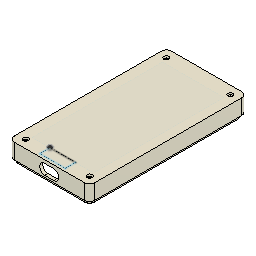
hk-case (Autodesk Fusion 360 design; units mm, degrees)
Autodesk Fusion 360 part; units mm, degrees
sketch "Base" plane through (0, 0, 0) normal (0, 1, 0) x (1, 0, 0)
  line L0 (26, -60) -> (-26, -60)
  line L1 (-30, -56) -> (-30, 56)
  line L2 (-26, 60) -> (26, 60)
  line L3 (30, 56) -> (30, -56)
  line L4 (30, -60) -> (-30, 60) construction
  line L5 (-30, -60) -> (30, 60) construction
  arc A0 (-26, 60) -> (-30, 56) centre (-26, 56) ccw
  arc A1 (30, 56) -> (26, 60) centre (26, 56) ccw
  arc A2 (-30, -56) -> (-26, -60) centre (-26, -56) ccw
  arc A3 (26, -60) -> (30, -56) centre (26, -56) ccw
  circle A4 centre (0, 0) radius 7.5
  line L6 (27.5, -61.5) -> (-27.5, -61.5)
  line L7 (-31.5, -57.5) -> (-31.5, 57.5)
  line L8 (-27.5, 61.5) -> (27.5, 61.5)
  line L9 (31.5, 57.5) -> (31.5, -57.5)
  line L10 (31.5, -61.5) -> (-31.5, 61.5) construction
  line L11 (-31.5, -61.5) -> (31.5, 61.5) construction
  arc A5 (-27.5, 61.5) -> (-31.5, 57.5) centre (-27.5, 57.5) ccw
  arc A6 (31.5, 57.5) -> (27.5, 61.5) centre (27.5, 57.5) ccw
  arc A7 (-31.5, -57.5) -> (-27.5, -61.5) centre (-27.5, -57.5) ccw
  arc A8 (27.5, -61.5) -> (31.5, -57.5) centre (27.5, -57.5) ccw
  circle A9 centre (-25, -55) radius 2.5
  circle A10 centre (25, -55) radius 2.5
  circle A11 centre (25, 55) radius 2.5
  circle A12 centre (-25, 55) radius 2.5
  circle A13 centre (-25, -55) radius 1.75
  circle A14 centre (25, -55) radius 1.75
  circle A15 centre (25, 55) radius 1.75
  circle A16 centre (-25, 55) radius 1.75
  circle A17 centre (-25, -55) radius 1
  circle A18 centre (25, -55) radius 1
  circle A19 centre (25, 55) radius 1
  circle A20 centre (-25, 55) radius 1
  circle A21 centre (-25, -55) radius 2
  circle A22 centre (25, -55) radius 2
  circle A23 centre (25, 55) radius 2
  circle A24 centre (-25, 55) radius 2
  line L12 (25, 59) -> (-25, 59)
  line L13 (-29, 55) -> (-29, -55)
  line L14 (-25, -59) -> (25, -59)
  line L15 (29, -55) -> (29, 55)
  line L16 (29, 59) -> (-29, -59) construction
  line L17 (-29, 59) -> (29, -59) construction
  arc A25 (25, -59) -> (29, -55) centre (25, -55) ccw
  arc A26 (-29, -55) -> (-25, -59) centre (-25, -55) ccw
  arc A27 (29, 55) -> (25, 59) centre (25, 55) ccw
  arc A28 (-25, 59) -> (-29, 55) centre (-25, 55) ccw
  dimension "d1" = 60
  dimension "d2" = 120
  dimension "d11" = 4
  dimension "d12" = 4
  dimension "d13" = 4
  dimension "d14" = 4
  dimension "d15" = 15
  dimension "d18" = 63
  dimension "d19" = 123
  dimension "d20" = 4
  dimension "d21" = 4
  dimension "d22" = 4
  dimension "d23" = 4
  dimension "d30" = 5
  dimension "d31" = 5
  dimension "d32" = 5
  dimension "d33" = 5
  dimension "d34" = 3.5
  dimension "d35" = 3.5
  dimension "d36" = 3.5
  dimension "d37" = 3.5
  dimension "d38" = 2
  dimension "d39" = 2
  dimension "d40" = 2
  dimension "d41" = 4
  dimension "d42" = 4
  dimension "d43" = 4
  dimension "d44" = 4
  dimension "d65" = 58
  dimension "d66" = 118
  dimension "d67" = 4
  dimension "d68" = 4
  dimension "d69" = 4
  dimension "d70" = 4
  constraint horizontal L0
  constraint perpendicular L0 L1
  constraint parallel L0 L2
  constraint parallel L1 L3
  constraint coincident L4 A4.centre
  constraint coincident L5 A4.centre
  constraint coincident A4.centre origin
  constraint coincident L4.end L2
  constraint coincident L4.end L1
  constraint tangent L2 A0
  constraint tangent L1 A0
  constraint coincident L5.end L2
  constraint coincident L5.end L3
  constraint tangent L2 A1
  constraint tangent L3 A1
  constraint coincident L5.start L1
  constraint coincident L5.start L0
  constraint tangent L1 A2
  constraint tangent L0 A2
  constraint coincident L4.start L0
  constraint coincident L4.start L3
  constraint tangent L0 A3
  constraint tangent L3 A3
  constraint horizontal L6
  constraint perpendicular L6 L7
  constraint parallel L6 L8
  constraint parallel L7 L9
  constraint coincident L10 A4.centre
  constraint coincident L11 A4.centre
  constraint coincident L10.end L8
  constraint coincident L10.end L7
  constraint tangent L8 A5
  constraint tangent L7 A5
  constraint coincident L11.end L8
  constraint coincident L11.end L9
  constraint tangent L8 A6
  constraint tangent L9 A6
  constraint coincident L11.start L7
  constraint coincident L11.start L6
  constraint tangent L7 A7
  constraint tangent L6 A7
  constraint coincident L10.start L6
  constraint coincident L10.start L9
  constraint tangent L6 A8
  constraint tangent L9 A8
  constraint concentric A9 A13
  constraint concentric A10 A14
  constraint concentric A11 A15
  constraint concentric A12 A16
  constraint concentric A9 A17
  constraint concentric A14 A18
  constraint concentric A11 A19
  constraint concentric A16 A20
  constraint concentric A13 A21
  constraint concentric A10 A22
  constraint concentric A15 A23
  constraint concentric A16 A24
  constraint horizontal L12
  constraint perpendicular L12 L13
  constraint parallel L12 L14
  constraint parallel L13 L15
  constraint coincident L16 A4.centre
  constraint coincident L17 A4.centre
  constraint coincident L17.end L14
  constraint coincident L17.end L15
  constraint tangent L14 A25
  constraint tangent L15 A25
  constraint coincident L16.end L14
  constraint coincident L16.end L13
  constraint tangent L14 A26
  constraint tangent L13 A26
  constraint coincident L16.start L15
  constraint coincident L16.start L12
  constraint tangent L15 A27
  constraint tangent L12 A27
  constraint coincident L17.start L13
  constraint coincident L17.start L12
  constraint tangent L13 A28
  constraint tangent L12 A28
  measures "d1" distance of L4.end L5.end
  measures "d2" distance of L5.start L4.end
  measures "d11" radius of A0
  measures "d12" radius of A1
  measures "d13" radius of A2
  measures "d14" radius of A3
  measures "d15" diameter of A4
  measures "d18" distance of L10.end L11.end
  measures "d19" distance of L11.start L10.end
  measures "d20" radius of A5
  measures "d21" radius of A6
  measures "d22" radius of A7
  measures "d23" radius of A8
  measures "d30" diameter of A9
  measures "d31" diameter of A10
  measures "d32" diameter of A11
  measures "d33" diameter of A12
  measures "d34" diameter of A13
  measures "d35" diameter of A14
  measures "d36" diameter of A15
  measures "d37" diameter of A16
  measures "d38" diameter of A17
  measures "d39" diameter of A19
  measures "d40" diameter of A20
  measures "d41" diameter of A21
  measures "d42" diameter of A22
  measures "d43" diameter of A23
  measures "d44" diameter of A24
  measures "d65" distance of L16.end L17.end
  measures "d66" distance of L17.start L16.end
  measures "d67" radius of A25
  measures "d68" radius of A26
  measures "d69" radius of A27
  measures "d70" radius of A28
extrude "Extrude2" add sketch "Base" against normal blind 4 contours L6 L7 L8 L9 A5 A6 A7 A8 makes body 1
extrude "Extrude3" add sketch "Base" against normal blind 2.5 contours L0 L1 L2 L3 A0 A1 A2 A3 | A4 | A9 | A10 | A11 | A12 | A13 | A14 | A15 | A16 | A21 | A22 | A23 | A24 | L12 L13 L14 L15 A25 A26 A27 A28 bodies 1
sketch "PCB Footprint" plane through (0, -2.5, 0) normal (0, -1, 0) x (1, 0, 0)
  arc A0 (-26, 60) -> (-30, 56) centre (-26, 56) ccw
  line L0 (-30, 56) -> (-30, -56)
  arc A1 (-30, -56) -> (-26, -60) centre (-26, -56) ccw
  line L1 (-26, -60) -> (26, -60)
  arc A2 (26, -60) -> (30, -56) centre (26, -56) ccw
  line L2 (30, -56) -> (30, 56)
  arc A3 (30, 56) -> (26, 60) centre (26, 56) ccw
  line L3 (26, 60) -> (-26, 60)
  line L4 (24, -51) -> (-24, -51)
  line L5 (-24, -51) -> (-24, 51)
  line L6 (-24, 51) -> (24, 51)
  line L7 (24, 51) -> (24, -51)
  line L8 (24, -51) -> (-24, 51) construction
  line L9 (-24, -51) -> (24, 51) construction
  circle A4 centre (25, -55) radius 1
  circle A5 centre (-25, -55) radius 1
  circle A6 centre (25, 55) radius 1
  circle A7 centre (-25, 55) radius 1
  line L10 (25, -52) -> (-25, -52)
  line L11 (-25, -52) -> (-25, 52)
  line L12 (-25, 52) -> (25, 52)
  line L13 (25, 52) -> (25, -52)
  line L14 (25, -52) -> (-25, 52) construction
  line L15 (-25, -52) -> (25, 52) construction
  dimension "d28" = 48
  dimension "d29" = 102
  dimension "d47" = 50
  dimension "d48" = 104
  constraint horizontal L4
  constraint perpendicular L4 L5
  constraint parallel L4 L6
  constraint parallel L5 L7
  constraint coincident L8 origin
  constraint coincident L9 origin
  constraint horizontal L10
  constraint perpendicular L10 L11
  constraint parallel L10 L12
  constraint parallel L11 L13
  constraint coincident L14 origin
  constraint coincident L15 origin
  measures "d28" distance of L5.end L6.end
  measures "d29" distance of L4.end L5.end
  measures "d47" distance of L11.end L12.end
  measures "d48" distance of L10.end L11.end
extrude "Extrude4" cut sketch "Base" against normal blind 1.5 contours A13 | A14 | A15 | A16 | A21 | A22 | A23 | A24 bodies 1
extrude "Extrude5" add sketch "PCB Footprint" along normal blind 2 contours L10 L11 L12 L13 bodies 1
fillet "Fillet1" radius 1 4 edges at (0, -2.5, 52) (25, -2.5, 0) (-25, -2.5, 0) (0, -2.5, -52) on bodies 1
extrude "Extrude6" add sketch "Base" along normal blind 5 separate body contours L6 L7 L8 L9 A5 A6 A7 A8 makes body 2
extrude "Extrude7" add sketch "Base" along normal blind 1.5 contours L0 L1 L2 L3 A0 A1 A2 A3 | A9 | A10 | A11 | A12 | A13 | A14 | A15 | A16 | A17 | A18 | A19 | A20 | A21 | A22 | A23 | A24 | L12 L13 L14 L15 A25 A26 A27 A28 bodies 2
extrude "Extrude8" add sketch "Base" along normal blind 3.5 contours A13 | A14 | A15 | A16 bodies 2
fillet "Fillet2" radius 2 4 edges at (-26.6316, 1.5, 54.3672) (23.3684, 1.5, 54.3672) (-26.6316, 1.5, -55.6328) (23.3684, 1.5, -55.6328) on bodies 2
copy_body "Body->Comp1" bodies 1 removing the originals makes body 3 in component "Bottom"
copy_body "Body->Comp2" bodies 2 removing the originals makes body 4 in component "Top"
extrude "Extrude1" add sketch "Base" against normal blind 15 contours L0 L1 L2 L3 A0 A1 A2 A3 bodies 3 in component "Bottom"
fillet "Fillet1'" radius 0.5 8 edges at (30, -15, 0) (28.8284, -15, 58.8284) (0, -15, 60) (-28.8284, -15, 58.8284) (-30, -15, 0) (-28.8284, -15, -58.8284) (0, -15, -60) (28.8284, -15, -58.8284) on bodies 3 in component "Bottom"
sketch "Sketch3" plane through (0, 1.5, 0) normal (0, 1, 0) x (-1, 0, 0)
  circle A0 centre (25, -55) radius 3.75
  circle A1 centre (25, 55) radius 3.75
  circle A2 centre (0, 0) radius 7.5
  arc A3 (30, 56) -> (26, 60) centre (26, 56) ccw
  line L0 (26, 60) -> (-26, 60)
  arc A4 (-26, 60) -> (-30, 56) centre (-26, 56) ccw
  line L1 (-30, 56) -> (-30, -56)
  arc A5 (-30, -56) -> (-26, -60) centre (-26, -56) ccw
  line L2 (-26, -60) -> (26, -60)
  arc A6 (26, -60) -> (30, -56) centre (26, -56) ccw
  line L3 (30, -56) -> (30, 56)
  circle A7 centre (-25, 55) radius 3.75
  circle A8 centre (-25, -55) radius 3.75
  line L4 (26.5, 60.5) -> (-26.5, 60.5)
  line L5 (-30.5, 56.5) -> (-30.5, -56.5)
  line L6 (-26.5, -60.5) -> (26.5, -60.5)
  line L7 (30.5, -56.5) -> (30.5, 56.5)
  line L8 (30.5, 60.5) -> (-30.5, -60.5) construction
  line L9 (-30.5, 60.5) -> (30.5, -60.5) construction
  arc A9 (26.5, -60.5) -> (30.5, -56.5) centre (26.5, -56.5) ccw
  arc A10 (-30.5, -56.5) -> (-26.5, -60.5) centre (-26.5, -56.5) ccw
  arc A11 (30.5, 56.5) -> (26.5, 60.5) centre (26.5, 56.5) ccw
  arc A12 (-26.5, 60.5) -> (-30.5, 56.5) centre (-26.5, 56.5) ccw
  dimension "d75" = 61
  dimension "d76" = 121
  dimension "d77" = 4
  dimension "d78" = 4
  dimension "d79" = 4
  dimension "d80" = 4
  constraint horizontal L4
  constraint perpendicular L4 L5
  constraint parallel L4 L6
  constraint parallel L5 L7
  constraint coincident L8 A2.centre
  constraint coincident L9 A2.centre
  constraint coincident A2.centre origin
  constraint coincident L9.end L6
  constraint coincident L9.end L7
  constraint tangent L6 A9
  constraint tangent L7 A9
  constraint coincident L8.end L6
  constraint coincident L8.end L5
  constraint tangent L6 A10
  constraint tangent L5 A10
  constraint coincident L8.start L7
  constraint coincident L8.start L4
  constraint tangent L7 A11
  constraint tangent L4 A11
  constraint coincident L9.start L4
  constraint coincident L9.start L5
  constraint tangent L4 A12
  constraint tangent L5 A12
  measures "d75" distance of L8.end L9.end
  measures "d76" distance of L9.start L8.end
  measures "d77" radius of A9
  measures "d78" radius of A10
  measures "d79" radius of A11
  measures "d80" radius of A12
extrude "Extrude2'" add 1 faces at (31, -4, 18.6667) along direction (0, -1, 0) blind 8 on bodies 3 bodies 3 in component "Bottom"
sketch "Sketch4" plane through (0, 0, 61.5) normal (0, 0, 1) x (1, 0, 0)
  line L0 (27.5, 0) -> (-27.5, 0)
  line L1 (-27.5, 0) -> (-27.5, -12)
  line L2 (-27.5, -12) -> (27.5, -12)
  line L3 (27.5, -12) -> (27.5, 0)
  line L4 (3.5, -10.5) -> (-3.5, -10.5)
  line L5 (-3.5, -2.5) -> (3.5, -2.5)
  arc A0 (-3.5, -2.5) -> (-7.5, -6.5) centre (-3.5, -6.5) ccw
  arc A1 (7.5, -6.5) -> (3.5, -2.5) centre (3.5, -6.5) ccw
  arc A2 (-7.5, -6.5) -> (-3.5, -10.5) centre (-3.5, -6.5) ccw
  arc A3 (3.5, -10.5) -> (7.5, -6.5) centre (3.5, -6.5) ccw
  dimension "d93" = 4
  dimension "d94" = 4
  dimension "d95" = 4
  dimension "d96" = 4
  constraint horizontal L4
  constraint parallel L4 L5
  constraint tangent L5 A0
  constraint tangent L5 A1
  constraint tangent L4 A2
  constraint coincident A0.end A2.start
  constraint tangent L4 A3
  constraint coincident A1.start A3.end
  measures "d93" radius of A0
  measures "d94" radius of A1
  measures "d95" radius of A2
  measures "d96" radius of A3
extrude "Extrude4'" cut sketch "Sketch4" against normal blind 3 contours L4 L5 A0 A1 A2 A3 bodies 3 in component "Bottom"
extrude "Extrude5'" cut 1 faces at (8, -2.5, 17) along direction (0, 1, 0) blind 2 on bodies 3 bodies 3 in component "Bottom"
sketch "Sketch5" plane through (0, -0.5, 0) normal (0, -1, 0) x (1, 0, 0)
  line L0 (-24, 51) -> (-24, -51)
  line L1 (-24, -51) -> (24, -51)
  line L2 (24, -51) -> (24, 51)
  line L3 (24, 51) -> (-24, 51)
  line L4 (-9.8896, 51) -> (10, 51)
  line L5 (10, 51) -> (10, 59)
  line L6 (10, 59) -> (-9.8896, 59)
  line L7 (-9.8896, 59) -> (-9.8896, 51)
  constraint horizontal L4
  constraint vertical L5
  constraint horizontal L6
  constraint vertical L7
  constraint coincident L3 L4.start
extrude "Extrude6'" cut sketch "Sketch5" along normal blind 4 contours L3 L4 L5 L6 L7 bodies 3 in component "Bottom"
extrude "Extrude7'" add sketch "Sketch5" along normal blind 1.5 contours L0 L1 L2 L3 L4 bodies 3 in component "Bottom"
other "Base Mesh Feature1"
component "Bottom" placed x (1, 0, 0) y (0, 1, 0) z (0, 0, 1) at (0, 0, 0)
component "Top" placed x (1, 0, 0) y (0, 1, 0) z (0, 0, 1) at (0, -9, 0)
named bodies: "Bottom", "Top"
